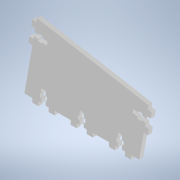
# Autodesk Inventor part: tc_support_down
Saved by Autodesk Inventor 2020.1 (Build 241239000, 239)
## iProperties
Created: 2019-07-16
Part Number: tc_support_down
Material: Acier inoxydable
Document SubType Name: Modeling
Designer: Thibault
Density: 8 g/cm^3
Appearance: Semi-poli
extra_height_front: 23,000 mm
extra_height_back: 13,108 mm
Author: Thibault
Autodesk Inventor part; units mm, degrees
ref_plane "YZ Plane" through (0, 0, 0) normal (1, 0, 0) x (0, 1, 0)
ref_plane "XZ Plane" through (0, 0, 0) normal (0, 1, 0) x (-1, 0, 0)
ref_plane "XY Plane" through (0, 0, 0) normal (0, 0, 1) x (1, 0, 0)
sketch "Anchor (screw side)" plane through (0, 0, 0) normal (0, 0, 1) x (1, 0, 0)
  circle A0 centre (93.7814, 50.2592) radius 1
  line L0 (91.2814, 51.2592) -> (88.2814, 51.2592)
  line L1 (88.2814, 51.2592) -> (88.2814, 49.2592)
  line L2 (88.2814, 49.2592) -> (91.2814, 49.2592)
  line L3 (91.2814, 49.2592) -> (91.2814, 51.2592)
  line L4 (99.2814, 51.2592) -> (96.2814, 51.2592)
  line L5 (96.2814, 51.2592) -> (96.2814, 49.2592)
  line L6 (96.2814, 49.2592) -> (99.2814, 49.2592)
  line L7 (99.2814, 49.2592) -> (99.2814, 51.2592)
  line L8 (91.2814, 51.2592) -> (96.2814, 49.2592) construction
  line L9 (96.2814, 51.2592) -> (91.2814, 49.2592) construction
  line L10 (86.2814, 53.2592) -> (101.2814, 53.2592) construction
  line L11 (101.2814, 53.2592) -> (101.2814, 47.2592) construction
  line L12 (101.2814, 47.2592) -> (86.2814, 47.2592) construction
  line L13 (86.2814, 47.2592) -> (86.2814, 53.2592) construction
  point P0 (103.5798, 50.1132)
  dimension "d27" = 2
  dimension "d28" = 3
  dimension "d29" = 2
  dimension "d30" = 3
  dimension "d32" = 5
  dimension "d34" = 2
  dimension "d35" = 2
  dimension "d36" = 2
  dimension "d37" = 2
  measures "d27" diameter of A0
  measures "d28" distance of L2.end L1.end
  measures "d29" distance of L1.end L0.end
  measures "d30" distance of L6.end L5.end
  measures "d32" distance between parallel lines of L5 L3
  measures "d34" distance between parallel lines of L0 L10
  measures "d35" distance between parallel lines of L12 L2
  measures "d36" distance between parallel lines of L11 L7
  measures "d37" distance between parallel lines of L13 L1
sketch "Anchor (nut side)" plane through (0, 0, 0) normal (0, 0, 1) x (1, 0, 0)
  line L0 (10, 0) -> (8.5, 0)
  line L1 (8.5, 0) -> (8.5, -2)
  line L2 (8.5, -2) -> (9.3, -2)
  line L3 (9.3, -2) -> (9.3, -4)
  line L4 (5.7, -4) -> (5.7, -2)
  line L5 (5.7, -2) -> (6.5, -2)
  line L6 (6.5, -2) -> (6.5, 0)
  line L7 (6.5, 0) -> (5, 0)
  line L8 (2, 0) -> (2, 2)
  line L9 (2, 0) -> (3, 0) construction
  line L10 (2, 2) -> (5, 2)
  line L11 (5, 2) -> (5, 0)
  line L12 (5, 2) -> (7, 2) construction
  line L13 (10, 0) -> (10, 2)
  line L14 (10, 2) -> (13, 2)
  line L15 (13, 2) -> (13, 0)
  line L16 (0, 0) -> (2, 0)
  line L17 (13, 0) -> (15, 0)
  line L18 (5.7, -4) -> (6.5, -4)
  line L19 (9.3, -4) -> (8.5, -4)
  line L20 (6.5, -4) -> (6.5, -6.25)
  line L21 (8.5, -4) -> (8.5, -6.25)
  line L22 (6.75, -6.5) -> (7.5, -6.5)
  arc A0 (6.5, -6.25) -> (6.75, -6.5) centre (6.75, -6.25) ccw
  arc A1 (8.25, -6.5) -> (8.5, -6.25) centre (8.25, -6.25) ccw
  line L23 (7.5, -7.2938) -> (7.5, -4.9797)
  line L24 (7.5, -6.5) -> (8.25, -6.5)
  point P0 (9.1321, -0.6227)
  point P1 (6.5, -6.5)
  point P2 (8.5, -6.5)
  dimension "d3" = 2
  dimension "d7" = 5
  dimension "d10" = 1.5
  dimension "d11" = 2
  dimension "d12" = 0.8
  dimension "d13" = 2
  dimension "d14" = 0.8
  dimension "d15" = 2
  dimension "d18" = 2
  dimension "d19" = 0.8
  dimension "d20" = 0.8
  dimension "d21" = 2.5
  dimension "d22" = 2.5
  dimension "d23" = 2
  dimension "d38" = 2
  dimension "d39" = 0.25
  dimension "d118" = 2
  dimension "d120" = 3
  measures "d3" distance of point (0, 0) L8.start
  measures "d7" distance of L7.end L0.start
  measures "d10" distance of L0.start L0.end
  measures "d11" distance of L0.end L1.end
  measures "d12" distance of L1.end L2.end
  measures "d13" distance of L2.end L3.end
  measures "d14" distance of L4.end L5.end
  measures "d15" distance of L6.end L0.end
  measures "d18" distance of L15.end point (15, 0)
  measures "d19" distance of L4.start L18.end
  measures "d20" distance of L3.end L19.end
  measures "d21" distance of L18.end point (6.5, -6.5)
  measures "d22" distance of L19.end point (8.5, -6.5)
  measures "d23" distance of L18.end L19.end
  measures "d38" distance of the line from the sketch origin of L10
  measures "d39" radius of A0
  measures "d118" distance between parallel lines of L0 L14
  measures "d120" distance of L8.end L10.end
derived "shared_parameters.ipt"
sketch "Esquisse2" plane through (0, 0, 0) normal (0, 0, 1) x (1, 0, 0)
  line L0 (-2.5952, 8.7856) -> (1.4048, 8.7856)
  line L1 (16.4048, 8.7856) -> (20.4048, 8.7856)
  line L2 (-17.5952, 8.7856) -> (-19.5779, 8.7856)
  line L3 (35.4048, 8.7856) -> (37.3875, 8.7856)
  line L4 (-19.5779, 8.7856) -> (-15.9313, 29.4666)
  line L5 (-13.3266, 44.2387) -> (41.9211, 34.497)
  line L6 (39.3164, 19.7249) -> (37.3875, 8.7856)
  line L7 (-12.5952, 8.7856) -> (-11.0952, 8.7856)
  line L8 (-11.0952, 8.7856) -> (-11.0952, 10.7856)
  line L9 (-11.0952, 10.7856) -> (-11.8952, 10.7856)
  line L10 (-11.8952, 10.7856) -> (-11.8952, 12.7856)
  line L11 (-8.2952, 12.7856) -> (-8.2952, 10.7856)
  line L12 (-8.2952, 10.7856) -> (-9.0952, 10.7856)
  line L13 (-9.0952, 10.7856) -> (-9.0952, 8.7856)
  line L14 (-9.0952, 8.7856) -> (-7.5952, 8.7856)
  line L15 (-4.5952, 8.7856) -> (-4.5952, 6.7856)
  line L16 (-4.5952, 8.7856) -> (-5.5952, 8.7856) construction
  line L17 (-4.5952, 6.7856) -> (-7.5952, 6.7856)
  line L18 (-7.5952, 6.7856) -> (-7.5952, 8.7856)
  line L19 (-7.5952, 6.7856) -> (-9.5952, 6.7856) construction
  line L20 (-12.5952, 8.7856) -> (-12.5952, 6.7856)
  line L21 (-12.5952, 6.7856) -> (-15.5952, 6.7856)
  line L22 (-15.5952, 6.7856) -> (-15.5952, 8.7856)
  line L23 (-2.5952, 8.7856) -> (-4.5952, 8.7856)
  line L24 (-15.5952, 8.7856) -> (-17.5952, 8.7856)
  line L25 (-8.2952, 12.7856) -> (-9.0952, 12.7856)
  line L26 (-11.8952, 12.7856) -> (-11.0952, 12.7856)
  line L27 (-9.0952, 12.7856) -> (-9.0952, 15.0356)
  line L28 (-11.0952, 12.7856) -> (-11.0952, 15.0356)
  line L29 (-9.3452, 15.2856) -> (-10.0952, 15.2856)
  arc A0 (-9.0952, 15.0356) -> (-9.3452, 15.2856) centre (-9.3452, 15.0356) ccw
  arc A1 (-10.8452, 15.2856) -> (-11.0952, 15.0356) centre (-10.8452, 15.0356) ccw
  line L30 (-10.0952, 16.0794) -> (-10.0952, 13.7654)
  line L31 (-10.0952, 15.2856) -> (-10.8452, 15.2856)
  line L32 (6.4048, 8.7856) -> (7.9048, 8.7856)
  line L33 (7.9048, 8.7856) -> (7.9048, 10.7856)
  line L34 (7.9048, 10.7856) -> (7.1048, 10.7856)
  line L35 (7.1048, 10.7856) -> (7.1048, 12.7856)
  line L36 (10.7048, 12.7856) -> (10.7048, 10.7856)
  line L37 (10.7048, 10.7856) -> (9.9048, 10.7856)
  line L38 (9.9048, 10.7856) -> (9.9048, 8.7856)
  line L39 (9.9048, 8.7856) -> (11.4048, 8.7856)
  line L40 (14.4048, 8.7856) -> (14.4048, 6.7856)
  line L41 (14.4048, 8.7856) -> (13.4048, 8.7856) construction
  line L42 (14.4048, 6.7856) -> (11.4048, 6.7856)
  line L43 (11.4048, 6.7856) -> (11.4048, 8.7856)
  line L44 (11.4048, 6.7856) -> (9.4048, 6.7856) construction
  line L45 (6.4048, 8.7856) -> (6.4048, 6.7856)
  line L46 (6.4048, 6.7856) -> (3.4048, 6.7856)
  line L47 (3.4048, 6.7856) -> (3.4048, 8.7856)
  line L48 (16.4048, 8.7856) -> (14.4048, 8.7856)
  line L49 (3.4048, 8.7856) -> (1.4048, 8.7856)
  line L50 (10.7048, 12.7856) -> (9.9048, 12.7856)
  line L51 (7.1048, 12.7856) -> (7.9048, 12.7856)
  line L52 (9.9048, 12.7856) -> (9.9048, 15.0356)
  line L53 (7.9048, 12.7856) -> (7.9048, 15.0356)
  line L54 (9.6548, 15.2856) -> (8.9048, 15.2856)
  arc A2 (9.9048, 15.0356) -> (9.6548, 15.2856) centre (9.6548, 15.0356) ccw
  arc A3 (8.1548, 15.2856) -> (7.9048, 15.0356) centre (8.1548, 15.0356) ccw
  line L55 (8.9048, 16.0794) -> (8.9048, 13.7654)
  line L56 (8.9048, 15.2856) -> (8.1548, 15.2856)
  line L57 (25.4048, 8.7856) -> (26.9048, 8.7856)
  line L58 (26.9048, 8.7856) -> (26.9048, 10.7856)
  line L59 (26.9048, 10.7856) -> (26.1048, 10.7856)
  line L60 (26.1048, 10.7856) -> (26.1048, 12.7856)
  line L61 (29.7048, 12.7856) -> (29.7048, 10.7856)
  line L62 (29.7048, 10.7856) -> (28.9048, 10.7856)
  line L63 (28.9048, 10.7856) -> (28.9048, 8.7856)
  line L64 (28.9048, 8.7856) -> (30.4048, 8.7856)
  line L65 (33.4048, 8.7856) -> (33.4048, 6.7856)
  line L66 (33.4048, 8.7856) -> (32.4048, 8.7856) construction
  line L67 (33.4048, 6.7856) -> (30.4048, 6.7856)
  line L68 (30.4048, 6.7856) -> (30.4048, 8.7856)
  line L69 (30.4048, 6.7856) -> (28.4048, 6.7856) construction
  line L70 (25.4048, 8.7856) -> (25.4048, 6.7856)
  line L71 (25.4048, 6.7856) -> (22.4048, 6.7856)
  line L72 (22.4048, 6.7856) -> (22.4048, 8.7856)
  line L73 (35.4048, 8.7856) -> (33.4048, 8.7856)
  line L74 (22.4048, 8.7856) -> (20.4048, 8.7856)
  line L75 (29.7048, 12.7856) -> (28.9048, 12.7856)
  line L76 (26.1048, 12.7856) -> (26.9048, 12.7856)
  line L77 (28.9048, 12.7856) -> (28.9048, 15.0356)
  line L78 (26.9048, 12.7856) -> (26.9048, 15.0356)
  line L79 (28.6548, 15.2856) -> (27.9048, 15.2856)
  arc A4 (28.9048, 15.0356) -> (28.6548, 15.2856) centre (28.6548, 15.0356) ccw
  arc A5 (27.1548, 15.2856) -> (26.9048, 15.0356) centre (27.1548, 15.0356) ccw
  line L80 (27.9048, 16.0794) -> (27.9048, 13.7654)
  line L81 (27.9048, 15.2856) -> (27.1548, 15.2856)
  line L82 (-14.1948, 39.3147) -> (-14.4553, 37.8374)
  line L83 (-14.4553, 37.8374) -> (-12.4857, 37.4902)
  line L84 (-12.4857, 37.4902) -> (-12.3468, 38.278)
  line L85 (-12.3468, 38.278) -> (-10.3771, 37.9307)
  line L86 (-11.0023, 34.3854) -> (-12.9719, 34.7327)
  line L87 (-12.9719, 34.7327) -> (-12.833, 35.5205)
  line L88 (-12.833, 35.5205) -> (-14.8026, 35.8678)
  line L89 (-14.8026, 35.8678) -> (-15.0631, 34.3906)
  line L90 (-15.584, 31.4362) -> (-17.5536, 31.7835)
  line L91 (-15.584, 31.4362) -> (-15.4104, 32.421) construction
  line L92 (-17.5536, 31.7835) -> (-17.0327, 34.7379)
  line L93 (-17.0327, 34.7379) -> (-15.0631, 34.3906)
  line L94 (-17.0327, 34.7379) -> (-16.6854, 36.7075) construction
  line L95 (-14.1948, 39.3147) -> (-16.1644, 39.662)
  line L96 (-16.1644, 39.662) -> (-15.6435, 42.6164)
  line L97 (-15.6435, 42.6164) -> (-13.6739, 42.2691)
  line L98 (-15.9313, 29.4666) -> (-15.584, 31.4362)
  line L99 (-13.6739, 42.2691) -> (-13.3266, 44.2387)
  line L100 (-11.0023, 34.3854) -> (-10.8634, 35.1732)
  line L101 (-10.3771, 37.9307) -> (-10.5161, 37.1429)
  line L102 (-10.8634, 35.1732) -> (-8.6475, 34.7825)
  line L103 (-10.5161, 37.1429) -> (-8.3003, 36.7521)
  line L104 (-8.3579, 34.9853) -> (-8.2277, 35.7239)
  arc A6 (-8.6475, 34.7825) -> (-8.3579, 34.9853) centre (-8.6041, 35.0287) ccw
  arc A7 (-8.0975, 36.4625) -> (-8.3003, 36.7521) centre (-8.3437, 36.5059) ccw
  line L105 (-7.4459, 35.5861) -> (-9.7249, 35.9879)
  line L106 (-8.2277, 35.7239) -> (-8.0975, 36.4625)
  line L107 (40.1846, 24.649) -> (40.4451, 26.1262)
  line L108 (40.4451, 26.1262) -> (38.4755, 26.4735)
  line L109 (38.4755, 26.4735) -> (38.3366, 25.6856)
  line L110 (38.3366, 25.6856) -> (36.367, 26.0329)
  line L111 (36.9921, 29.5782) -> (38.9617, 29.2309)
  line L112 (38.9617, 29.2309) -> (38.8228, 28.4431)
  line L113 (38.8228, 28.4431) -> (40.7924, 28.0958)
  line L114 (40.7924, 28.0958) -> (41.0529, 29.573)
  line L115 (41.5738, 32.5274) -> (43.5434, 32.1801)
  line L116 (41.5738, 32.5274) -> (41.4002, 31.5426) construction
  line L117 (43.5434, 32.1801) -> (43.0225, 29.2257)
  line L118 (43.0225, 29.2257) -> (41.0529, 29.573)
  line L119 (43.0225, 29.2257) -> (42.6752, 27.2561) construction
  line L120 (40.1846, 24.649) -> (42.1543, 24.3017)
  line L121 (42.1543, 24.3017) -> (41.6333, 21.3472)
  line L122 (41.6333, 21.3472) -> (39.6637, 21.6945)
  line L123 (41.9211, 34.497) -> (41.5738, 32.5274)
  line L124 (39.6637, 21.6945) -> (39.3164, 19.7249)
  line L125 (36.9921, 29.5782) -> (36.8532, 28.7904)
  line L126 (36.367, 26.0329) -> (36.5059, 26.8208)
  line L127 (36.8532, 28.7904) -> (34.6374, 29.1811)
  line L128 (36.5059, 26.8208) -> (34.2901, 27.2115)
  line L129 (34.3478, 28.9783) -> (34.2175, 28.2397)
  arc A8 (34.6374, 29.1811) -> (34.3478, 28.9783) centre (34.594, 28.9349) ccw
  arc A9 (34.0873, 27.5011) -> (34.2901, 27.2115) centre (34.3335, 27.4577) ccw
  line L130 (33.4358, 28.3775) -> (35.7147, 27.9757)
  line L131 (34.2175, 28.2397) -> (34.0873, 27.5011)
  point P0 (0, 0)
  point P1 (1.4048, 8.7856)
  point P2 (41.4613, 8.4849)
  point P3 (41.9211, 34.497)
  point P4 (-13.3266, 44.2387)
  point P5 (-17.8871, 8.2607)
  point P6 (39.7911, 6.6105)
  point P7 (-17.9917, 8.6071)
  dimension "d1" = 8
  dimension "d2" = 8
  dimension "d40" = 36
  dimension "d41" = 56.1
  dimension "d44" = 80
  dimension "extra_height_front" = 23
  dimension "extra_height_back" = 13.1081
  constraints: 14 end point, 5 horizontal, 1 collinear, 14 other
  measures "d41" distance of L5.end L5.start
  measures "d44" angle of L2 L4
extrude "Extrusion1" add sketch "Esquisse2" along normal blind 2
equation "\"d41\" = tc_base_support_dist"
equation "\"d31\" = sheet_thickness"
equation "\"tc_base_support_dist\" = 56.1"
equation "\"sheet_thickness\" = 2"
